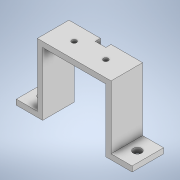
# Autodesk Inventor part: Door_motor_bracket
Saved by Autodesk Inventor 2020 (Build 240168000, 168)
## iProperties
Created: 2019-09-27
Part Number: Door_motor_bracket
Material: 일반
Document SubType Name: Modeling
Designer: Knowblesse
Density: 1 g/cm^3
Appearance: 기본값
Author: Knowblesse
## iProperties of the stored document _3D 인쇄.ipt
Created: 2019-09-27
Part Number: _3D 인쇄
Material: 일반
Document SubType Name: Modeling
Designer: Knowblesse
Density: 1 g/cm^3
Appearance: 기본값
Author: Knowblesse
Autodesk Inventor part; units mm, degrees
ref_plane "YZ Plane" through (0, 0, 0) normal (1, 0, 0) x (0, 1, 0)
ref_plane "XZ Plane" through (0, 0, 0) normal (0, 1, 0) x (-1, 0, 0)
ref_plane "XY Plane" through (0, 0, 0) normal (0, 0, 1) x (1, 0, 0)
sketch "스케치1" plane through (0, 0, 0) normal (0, 0, 1) x (1, 0, 0)
  line L0 (0, 0) -> (70, 0)
  line L1 (70, 0) -> (70, 65)
  line L2 (70, 65) -> (0, 65)
  line L3 (0, 65) -> (0, 0)
  line L4 (5, 0) -> (65, 0)
  line L5 (65, 0) -> (65, 60)
  line L6 (65, 60) -> (5, 60)
  line L7 (5, 60) -> (5, 0)
  line L8 (0, 0) -> (-20, 0)
  line L9 (-20, 0) -> (-20, 5)
  line L10 (-20, 5) -> (0, 5)
  line L11 (0, 5) -> (0, 0)
  line L12 (70, 0) -> (90, 0)
  line L13 (90, 0) -> (90, 5)
  line L14 (90, 5) -> (70, 5)
  line L15 (70, 5) -> (70, 0)
  dimension "d0" = 60
  dimension "d1" = 60
  dimension "d2" = 5
  dimension "d3" = 5
  dimension "d4" = 5
  dimension "d5" = 20
  dimension "d6" = 5
  dimension "d7" = 20
  dimension "d8" = 5
  constraints: 32 end point, 8 parallel, 4 horizontal, 4 perpendicular, 1 point on line
  measures "d0" distance between parallel lines of L0 L6
  measures "d1" distance between parallel lines of L5 L7
  measures "d2" distance between parallel lines of L2 L6
  measures "d3" distance between parallel lines of L5 L1
  measures "d4" distance between parallel lines of L3 L7
  measures "d5" distance of L9.end L10.end
  measures "d6" distance of L8.end L9.end
  measures "d7" distance of L14.end L13.end
  measures "d8" distance of L13.end L12.end
extrude "돌출1" add sketch "스케치1" along normal blind 30 contours L3 L2 L1 L0 L5 L6 L7 | L8 L9 L10 L3 | L1 L14 L13 L12
sketch "스케치2" plane through (70, 5, 0) normal (0, 1, 0) x (1, 0, 0)
  line L0 (-90, 0) -> (-90, -30) projected
  line L1 (20, 0) -> (20, -30) projected
  line L2 (-70, 0) -> (-70, -30) projected
  line L3 (0, 0) -> (0, -30) projected
  point P0 (-80, -15)
  point P1 (10, -15)
  dimension "d11" = 10
  dimension "d14" = 10
  measures "d11" distance from line of point (-80, -15) L0
  measures "d14" distance from line of point (10, -15) L3
hole "구멍1" at (-10, 5, 15) at (80, 5, 15) direction (0, -1, 0) diameter 8 end through all
sketch "스케치3" plane through (0, 65, 0) normal (0, 1, 0) x (1, 0, 0)
  line L0 (70, 0) -> (0, 0) projected
  line L1 (0, 0) -> (0, -30) projected
  line L2 (70, -30) -> (0, -30) projected
  line L3 (70, 0) -> (70, -30) projected
  line L4 (0, 0) -> (0, -30) projected
  point P0 (0, -15)
  point P1 (35, -30)
  point P2 (20, -15)
  point P3 (50, -15)
  point P4 (0, -15)
  dimension "d33" = 20
  dimension "d34" = 20
  constraints: 3 midpoint, 2 horizontal alignment
  measures "d33" distance of point (0, -15) point (20, -15)
  measures "d34" distance from line of L3 point (50, -15)
hole "구멍2" at (20, 65, 15) at (50, 65, 15) direction (0, -1, 0) diameter 4.6 end through all
sketch "스케치4" plane through (0, 65, 0) normal (0, 1, 0) x (1, 0, 0)
  line L0 (70, 0) -> (0, 0) projected
  line L1 (0, 0) -> (0, -30) projected
  line L2 (70, -30) -> (0, -30) projected
  line L3 (70, 0) -> (70, -30) projected
  line L4 (5, 0) -> (65, 0) projected
  line L5 (30, 0) -> (40, 0)
  line L6 (40, 0) -> (40, -5)
  line L7 (40, -5) -> (30, -5)
  line L8 (30, -5) -> (30, 0)
  point P0 (0, 0)
  point P1 (35, -5)
  point P2 (40, 0)
  dimension "d29" = 10
  dimension "d30" = 5
  constraints: 8 end point, 2 parallel, 1 horizontal, 1 midpoint, 1 perpendicular, 1 point on line
  measures "d29" distance of L6.end L7.end
  measures "d30" distance of L5.end L6.end
extrude "돌출2" cut sketch "스케치4" against normal blind 10 contours L6 L7 L8 L0
equation "\"d14\" = d13"
equation "\"d13\" = d11"
